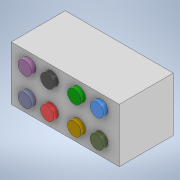
# Autodesk Inventor part: TreasureChestFinal
Saved by Autodesk Inventor 2021 (Build 250183000, 183)
## iProperties
Created: 2021-03-02
Part Number: TreasureChestFinal
Material: Generic
Document SubType Name: Modeling
Designer: con_c_000
Density: 1 g/cm^3
Appearance: Default
Author: con_c_000
Autodesk Inventor part; units mm, degrees
ref_plane "YZ Plane" through (0, 0, 0) normal (1, 0, 0) x (0, 1, 0)
ref_plane "XZ Plane" through (0, 0, 0) normal (0, 1, 0) x (-1, 0, 0)
ref_plane "XY Plane" through (0, 0, 0) normal (0, 0, 1) x (1, 0, 0)
sketch "Sketch1" plane through (0, 0, 0) normal (0, 1, 0) x (-1, 0, 0)
  line L0 (9.1659, 4.2179) -> (-600.4341, 4.2179)
  line L1 (-600.4341, 4.2179) -> (-600.4341, -300.5821)
  line L2 (-600.4341, -300.5821) -> (9.1659, -300.5821)
  line L3 (9.1659, -300.5821) -> (9.1659, 4.2179)
  point P0 (0, 0)
  dimension "d0" = 609.6
  dimension "d1" = 304.8
  constraints: 8 end point, 2 parallel, 1 horizontal, 1 perpendicular
  measures "d0" distance of L2.end L1.end
  measures "d1" distance of L1.end L0.end
extrude "Extrusion1" add sketch "Sketch1" along normal blind 304.8
sketch "Sketch2" plane through (-9.1659, 0, 4.2179) normal (0, 0, 1) x (1, 0, 0)
  circle A0 centre (101.6, 83.5824) radius 38.1
  circle A1 centre (228.6, 83.5824) radius 38.1
  circle A2 centre (381, 83.5824) radius 38.1
  circle A3 centre (508, 83.5824) radius 38.1
  circle A4 centre (508, 240.9926) radius 38.1
  circle A5 centre (381, 240.9926) radius 38.1
  circle A6 centre (228.6, 240.9926) radius 38.1
  circle A7 centre (101.6, 240.9926) radius 38.1
  line L0 (609.6, 0) -> (609.6, 304.8) projected
  line L1 (0, 0) -> (0, 304.8) projected
  point P0 (9.1659, 0)
  dimension "d4" = 76.2
  dimension "d5" = 76.2
  dimension "d6" = 76.2
  dimension "d7" = 76.2
  dimension "d8" = 76.2
  dimension "d9" = 76.2
  dimension "d10" = 76.2
  dimension "d11" = 76.2
  dimension "d12" = 101.6
  dimension "d13" = 127
  dimension "d14" = 101.6
  dimension "d15" = 127
  constraints: 8 centre point
  measures "d4" diameter of A0
  measures "d5" diameter of A1
  measures "d6" diameter of A2
  measures "d7" diameter of A3
  measures "d8" diameter of A4
  measures "d9" diameter of A5
  measures "d10" diameter of A6
  measures "d11" diameter of A7
  measures "d12" distance from line of L0 A4.centre
  measures "d13" distance of A4.centre A5.centre
  measures "d14" distance from line of L1 A7.centre
  measures "d15" distance of A7.centre A6.centre
extrude "Extrusion2" add sketch "Sketch2" along normal blind 25.4
body "Solid1"
